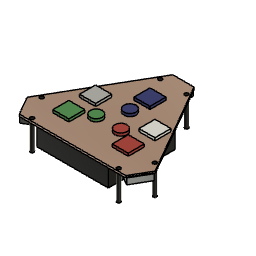
HyperShades Console mk.2 (Autodesk Fusion 360 design; units mm, degrees)
Autodesk Fusion 360 part; units mm, degrees
sketch "Board Sketch" plane through (0, 0, 0) normal (0, 0, 1) x (1, 0, 0)
  line L0 (0, 96.8013) -> (-55.8882, 0)
  line L1 (-55.8882, 0) -> (55.8882, 0)
  line L2 (55.8882, 0) -> (0, 96.8013)
  line L3 (-8, 82.9449) -> (8, 82.9449)
  line L4 (39.8882, 0) -> (47.8882, 13.8564)
  line L5 (-39.8882, 0) -> (-47.8882, 13.8564)
  line L6 (25, 0) -> (-25, 0)
  line L7 (-25, 0) -> (-25, 53.5) construction
  line L8 (-25, 53.5) -> (25, 53.5) construction
  line L9 (25, 53.5) -> (25, 0) construction
  line L10 (25, 0) -> (-25, 53.5) construction
  line L11 (-25, 0) -> (25, 53.5) construction
  line L12 (-226.0461, 90.0559) -> (-326.0461, 90.0559)
  line L13 (-326.0461, 90.0559) -> (-326.0461, 200.0559)
  line L14 (-326.0461, 200.0559) -> (-226.0461, 200.0559)
  line L15 (-226.0461, 200.0559) -> (-226.0461, 90.0559)
  line L16 (-226.0461, 90.0559) -> (-326.0461, 200.0559) construction
  line L17 (-326.0461, 90.0559) -> (-226.0461, 200.0559) construction
  point P0 (0, 26.75)
  point P1 (-276.0461, 145.0559)
  dimension "d14" = 16
  dimension "d15" = 16
  dimension "d16" = 60
  dimension "d17" = 16
  dimension "d18" = 60
  dimension "d28" = 50
  dimension "d29" = 53.5
  dimension "d30" = 100
  dimension "d31" = 110
  constraint horizontal L1
  constraint equal L1 L2
  constraint equal L0 L1
  constraint vertical origin L0.start
  constraint horizontal origin L1.end
  constraint coincident L0 L3.start
  constraint coincident L2 L3.end
  constraint horizontal L3
  constraint coincident L1 L4.start
  constraint coincident L2 L4.end
  constraint coincident L1 L5.start
  constraint coincident L0 L5.end
  constraint horizontal L6
  constraint perpendicular L6 L7
  constraint parallel L6 L8
  constraint parallel L7 L9
  constraint coincident L10 P0
  constraint coincident L11 P0
  constraint vertical origin P0
  constraint coincident L2 L8.end
  constraint coincident origin L6
  constraint horizontal L12
  constraint perpendicular L12 L13
  constraint parallel L12 L14
  constraint parallel L13 L15
  constraint coincident L16 P1
  constraint coincident L17 P1
  measures "d14" distance of L3.start L3.end
  measures "d15" distance of L4.start L4.end
  measures "d16" angle of L1 L4
  measures "d17" distance of L5.start L5.end
  measures "d18" angle of L1 L5
  measures "d28" distance of L7.end L8.end
  measures "d29" distance of L6.end L7.end
  measures "d30" distance of L13.end L14.end
  measures "d31" distance of L12.end L13.end
extrude "Extrude1" add sketch "Board Sketch" along normal blind 1.6 contours L0 L1 L2 L3 L4 L5 L6 makes body 1
sketch "Components Sketch" plane through (0, 0, 1.6) normal (0, 0, 1) x (-1, 0, 0)
  line L0 (-39.8882, 0) -> (-47.8882, -13.8564)
  line L1 (-47.8882, -13.8564) -> (-8, -82.9449)
  line L2 (-8, -82.9449) -> (8, -82.9449)
  line L3 (8, -82.9449) -> (47.8882, -13.8564)
  line L4 (47.8882, -13.8564) -> (39.8882, 0)
  line L5 (39.8882, 0) -> (-39.8882, 0)
  line L6 (-40.1382, -0.433) -> (-27.1479, -7.933)
  line L7 (-27.1479, -7.933) -> (-34.6479, -20.9234)
  line L8 (-34.6479, -20.9234) -> (-47.6382, -13.4234)
  line L9 (-30.8979, -14.4282) -> (-43.8882, -6.9282) construction
  line L10 (-26.75, 0) -> (26.75, 0) construction
  line L11 (26.75, 0) -> (26.75, -50) construction
  line L12 (26.75, -50) -> (-26.75, -50) construction
  line L13 (-26.75, -50) -> (-26.75, 0) construction
  line L14 (-26.75, 0) -> (26.75, -50) construction
  line L15 (26.75, 0) -> (-26.75, -50) construction
  line L16 (7.5, -82.9449) -> (-7.5, -82.9449)
  line L17 (-7.5, -82.9449) -> (-7.5, -67.9449)
  line L18 (-7.5, -67.9449) -> (7.5, -67.9449)
  line L19 (7.5, -67.9449) -> (7.5, -82.9449)
  line L20 (0, -25) -> (0, 0) construction
  line L21 (27.1479, -7.933) -> (34.6479, -20.9234)
  line L22 (40.1382, -0.433) -> (27.1479, -7.933)
  line L23 (34.6479, -20.9234) -> (47.6382, -13.4234)
  circle A0 centre (-9.2472, -26.9282) radius 4.5
  circle A1 centre (9.2472, -26.9282) radius 4.5
  circle A2 centre (0, -42.9449) radius 4.5
  line L24 (-28.2376, -13.4282) -> (-16.2376, -13.4282)
  line L25 (-16.2376, -13.4282) -> (-16.2376, -25.4282)
  line L26 (-16.2376, -25.4282) -> (-28.2376, -25.4282)
  line L27 (-28.2376, -25.4282) -> (-28.2376, -13.4282)
  line L28 (-28.2376, -13.4282) -> (-16.2376, -25.4282) construction
  line L29 (-16.2376, -13.4282) -> (-28.2376, -25.4282) construction
  line L30 (-6, -51.9449) -> (6, -51.9449)
  line L31 (6, -51.9449) -> (6, -63.9449)
  line L32 (6, -63.9449) -> (-6, -63.9449)
  line L33 (-6, -63.9449) -> (-6, -51.9449)
  line L34 (-6, -51.9449) -> (6, -63.9449) construction
  line L35 (6, -51.9449) -> (-6, -63.9449) construction
  line L36 (16.2376, -13.4282) -> (16.2376, -25.4282)
  line L37 (16.2376, -25.4282) -> (28.2376, -25.4282)
  line L38 (28.2376, -25.4282) -> (28.2376, -13.4282)
  line L39 (28.2376, -13.4282) -> (16.2376, -13.4282)
  line L40 (-28.2376, -33.4282) -> (-16.2376, -33.4282)
  line L41 (-16.2376, -33.4282) -> (-16.2376, -45.4282)
  line L42 (-16.2376, -45.4282) -> (-28.2376, -45.4282)
  line L43 (-28.2376, -45.4282) -> (-28.2376, -33.4282)
  line L44 (-28.2376, -33.4282) -> (-16.2376, -45.4282) construction
  line L45 (-16.2376, -33.4282) -> (-28.2376, -45.4282) construction
  line L46 (28.2376, -33.4282) -> (16.2376, -33.4282)
  line L47 (16.2376, -33.4282) -> (16.2376, -45.4282)
  line L48 (28.2376, -45.4282) -> (28.2376, -33.4282)
  line L49 (16.2376, -45.4282) -> (28.2376, -45.4282)
  point P0 (-43.8882, -6.9282)
  point P1 (-30.8979, -14.4282)
  point P2 (0, -25)
  point P3 (0, -67.9449)
  point P4 (-22.2376, -19.4282)
  point P5 (0, -57.9449)
  point P6 (-22.2376, -39.4282)
  dimension "d32" = 15
  dimension "d33" = 15
  dimension "d34" = 90
  dimension "d35" = 53.5
  dimension "d36" = 50
  dimension "d37" = 15
  dimension "d38" = 15
  dimension "d39" = 9
  dimension "d40" = 40
  dimension "d41" = 9
  dimension "d42" = 40
  dimension "d43" = 12
  dimension "d44" = 12
  dimension "d45" = 25
  dimension "d46" = 12
  dimension "d47" = 12
  dimension "d48" = 25
  dimension "d49" = 12
  dimension "d50" = 12
  dimension "d51" = 20
  constraint coincident L0 L6.start
  constraint perpendicular L0 L6
  constraint perpendicular L6 L7
  constraint coincident L0 L8.end
  constraint perpendicular L0 L8
  constraint midpoint L0 P0
  constraint midpoint L7 P1
  constraint coincident P1 L9.start
  constraint coincident P0 L9.end
  constraint horizontal L10
  constraint perpendicular L10 L11
  constraint parallel L10 L12
  constraint parallel L11 L13
  constraint coincident L14 P2
  constraint coincident L15 P2
  constraint vertical L20.end P2
  constraint coincident L20.end L10
  constraint horizontal L16
  constraint vertical L17
  constraint horizontal L18
  constraint vertical L19
  constraint coincident L2 L16.start
  constraint midpoint L18 P3
  constraint vertical P2 P3
  constraint coincident P2 L20.start
  constraint coincident L20.end origin
  constraint symmetric L6.start L20 L22.start
  constraint symmetric L6.end L20 L21.start
  constraint symmetric L7.end L20 L21.end
  constraint symmetric L8.end L20 L23.end
  constraint collinear P0 P1 A0.centre
  constraint symmetric L20 A0 A1
  constraint vertical L20.end A2.centre
  constraint horizontal L24
  constraint perpendicular L24 L25
  constraint parallel L24 L26
  constraint parallel L25 L27
  constraint coincident L28 P4
  constraint coincident L29 P4
  constraint collinear P0 P1 P4
  constraint horizontal L30
  constraint perpendicular L30 L31
  constraint parallel L30 L32
  constraint parallel L31 L33
  constraint coincident L34 P5
  constraint coincident L35 P5
  constraint vertical L20.end P5
  constraint symmetric L20 L24.start L38.end
  constraint symmetric L20 L24.end L36.start
  constraint symmetric L20 L25.end L36.end
  constraint symmetric L20 L26.end L37.end
  constraint horizontal L40
  constraint perpendicular L40 L41
  constraint parallel L40 L42
  constraint parallel L41 L43
  constraint coincident L44 P6
  constraint coincident L45 P6
  constraint vertical P4 P6
  constraint symmetric L20 L40.start L46.start
  constraint symmetric L20 L40.end L46.end
  constraint symmetric L20 L41.end L47.end
  constraint symmetric L20 L42.end L48.start
  measures "d32" distance of L6.start L6.end
  measures "d33" distance of L6.end L7.end
  measures "d34" angle of L0 L9
  measures "d35" distance of L11.end L12.end
  measures "d36" distance of L10.end L11.end
  measures "d37" distance of L16.start L16.end
  measures "d38" distance of L16.start L18.end
  measures "d39" diameter of A0
  measures "d40" distance of P0 A0.centre
  measures "d41" diameter of A2
  measures "d42" distance of L16 A2.centre
  measures "d43" distance of L25.end L26.end
  measures "d44" distance of L24.end L25.end
  measures "d45" distance of P0 P4
  measures "d46" distance of L31.end L32.end
  measures "d47" distance of L30.end L31.end
  measures "d48" distance of L16 P5
  measures "d49" distance of L41.end L42.end
  measures "d50" distance of L40.end L41.end
  measures "d51" distance of P4 P6
extrude "Extrude2" add sketch "Components Sketch" along normal blind 2 separate body contours A0 | A1 | A2 | L24 L25 L26 L27 | L30 L31 L32 L33 | L36 L37 L38 L39 | L40 L41 L42 L43 | L46 L47 L48 L49 makes body 2 at (-20.2376, 41.4282, 1.6) makes body 3 at (-8.4473, 23.8608, 1.6) makes body 4 at (7.764, 27.5889, 1.6) makes body 5 at (-20.2376, 17.4282, 1.6) makes body 6 at (0.3338, 46.0972, 1.6) makes body 7 at (24.2376, 17.4282, 1.6) makes body 8 at (24.2376, 37.4282, 1.6) makes body 9 at (2, 55.9449, 1.6)
sketch "Battery Holder Sketch" plane through (0, 0, 0) normal (0, 0, -1) x (1, 0, 0)
  line L0 (47.8882, -13.8564) -> (39.8882, 0)
  line L1 (39.8882, 0) -> (-39.8882, 0)
  line L2 (-39.8882, 0) -> (-47.8882, -13.8564)
  line L3 (-47.8882, -13.8564) -> (-8, -82.9449)
  line L4 (-8, -82.9449) -> (8, -82.9449)
  line L5 (8, -82.9449) -> (47.8882, -13.8564)
  line L6 (26.75, -50) -> (26.75, 0)
  line L7 (-26.75, 0) -> (-26.75, -50)
  line L8 (-26.75, -50) -> (26.75, -50)
  line L9 (26.75, 0) -> (-26.75, 0)
extrude "Extrude3" add sketch "Battery Holder Sketch" along normal blind 13 separate body contours L1 L6 L7 L8 L9 makes body 10
sketch "Standoff Sketch" plane through (0, 0, 1.6) normal (0, 0, 1) x (-1, 0, 0)
  line L0 (39.8882, 0) -> (-39.8882, 0)
  line L1 (-39.8882, 0) -> (-47.8882, -13.8564)
  line L2 (-47.8882, -13.8564) -> (-8, -82.9449)
  line L3 (-8, -82.9449) -> (8, -82.9449)
  line L4 (8, -82.9449) -> (47.8882, -13.8564)
  line L5 (47.8882, -13.8564) -> (39.8882, 0)
  circle A0 centre (-9.85, -75.4449) radius 1.375
  circle A1 centre (-42.318, -19.2086) radius 1.375
  line L6 (-30.8979, -14.4282) -> (-43.8882, -6.9282) construction
  circle A2 centre (-32.468, -2.1479) radius 1.375
  line L7 (0, 0) -> (0, -67.9449) construction
  circle A3 centre (9.85, -75.4449) radius 1.375
  circle A4 centre (42.318, -19.2086) radius 1.375
  circle A5 centre (32.468, -2.1479) radius 1.375
  point P0 (-7.5, -75.4449)
  point P1 (-41.143, -17.1734)
  point P2 (-33.643, -4.183)
  dimension "d56" = 2.75
  dimension "d57" = 2.35
  dimension "d58" = 2.75
  dimension "d59" = 2.35
  dimension "d60" = 15
  constraint horizontal P0 A0.centre
  constraint collinear P1 P2 A1.centre
  constraint symmetric A1 L6 A2
  constraint coincident L7.start origin
  constraint symmetric A0 L7 A3
  constraint symmetric A1 L7 A4
  constraint symmetric A2 L7 A5
  measures "d56" diameter of A0
  measures "d57" distance of P0 A0.centre
  measures "d58" diameter of A1
  measures "d59" distance of P1 A1.centre
  measures "d60" distance of L6.start L6.end
extrude "Extrude4" cut sketch "Standoff Sketch" against normal up to surface (1.6 mm away) contours A0 | A1 | A2 | A3 | A4 | A5 bodies 1
sketch "Sketch6" plane through (0, 0, 1.6) normal (0, 0, 1) x (-1, 0, 0)
  circle A0 centre (42.318, -19.2086) radius 1.375
  circle A1 centre (-32.468, -2.1479) radius 1.375
  circle A2 centre (9.85, -75.4449) radius 1.375
  circle A3 centre (32.468, -2.1479) radius 1.375
  circle A4 centre (-42.318, -19.2086) radius 1.375
  circle A5 centre (-9.85, -75.4449) radius 1.375
  line L0 (-39.8882, 0) -> (-47.8882, -13.8564)
  line L1 (-47.8882, -13.8564) -> (-8, -82.9449)
  line L2 (-8, -82.9449) -> (8, -82.9449)
  line L3 (8, -82.9449) -> (47.8882, -13.8564)
  line L4 (47.8882, -13.8564) -> (39.8882, 0)
  line L5 (39.8882, 0) -> (-39.8882, 0)
extrude "Extrude5" add sketch "Sketch6" against normal blind 21.6 separate body contours A0 | A1 | A2 | A3 | A4 | A5 makes body 11 at (-40.9856, 19.5478, -12.8) makes body 12 at (31.0948, 2.2164, -12.8) makes body 13 at (11.0233, 76.1618, -12.8) makes body 14 at (-32.0301, 3.4513, -5.6) makes body 15 at (43.6505, 19.5478, -12.8) makes body 16 at (-11.0233, 76.1618, -12.8)
extrude "Extrude6" add sketch "Components Sketch" against normal blind 5.1 separate body contours L0 L6 L7 L8 | L4 L21 L22 L23 | L2 L16 L17 L18 L19 makes body 17 at (33.978, 9.7631, 1.6) makes body 18 at (-33.978, 9.7631, 1.6) makes body 19 at (2.5, 72.9449, 1.6)
move_body "Move1" bodies 17 19 18 to x (1, 0, 0) y (0, 1, 0) z (0, 0, 1) at (0, 0, -1)
equation "d63 = -20 mm - 1.6 mm"
equation "d65 = -1.6 mm - 3.5 mm"
named bodies: "Console PCB", "Battery Holder", "Short Button", "G LED", "R LED", "G Button", "B LED", "R Button", "Long Button", "B Button", "Standoff", "Standoff (1)", "Standoff (2)", "Standoff (3)", "Standoff (4)", "Standoff (5)"
